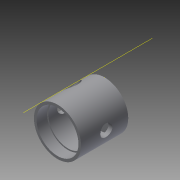
# Autodesk Inventor part: Piston
Saved by Autodesk Inventor 2015 (Build 190159000, 159)
## iProperties
Created: 2016-02-14
Part Number: Piston
Material: Generic
Document SubType Name: Modeling
Designer: Owner
Density: 1 g/cm^3
Appearance: Default
Author: Owner
Autodesk Inventor part; units mm, degrees
ref_plane "YZ Plane" through (0, 0, 0) normal (1, 0, 0) x (0, 1, 0)
ref_plane "XZ Plane" through (0, 0, 0) normal (0, 1, 0) x (-1, 0, 0)
ref_plane "XY Plane" through (0, 0, 0) normal (0, 0, 1) x (1, 0, 0)
sketch "Sketch1" plane through (0, 0, 0) normal (0, 0, 1) x (1, 0, 0)
  circle A0 centre (0, 0) radius 6.858
  dimension "d0" = 13.716
  constraints: 1 centre point, 1 coincident
  measures "d0" diameter of A0
extrude "Extrusion1" add sketch "Sketch1" along normal blind 13.716
hole "Hole1" at (0, 0, 13.716) direction (0, 0, -1) diameter 12.192 depth 3.048
hole "Hole2" at (0, 0, 10.668) direction (0, 0, -1) diameter 11.43 depth 9.144
sketch "Sketch2" plane through (0, 0, 0) normal (1, 0, 0) x (0, 1, 0)
  line L0 (0, 0) -> (0, 6.35)
  circle A0 centre (0, 6.35) radius 1.7399
  dimension "d21" = 6.35
  dimension "d22" = 3.4798
  constraints: 2 end point, 1 centre point, 1 coincident, 1 vertical
  measures "d21" distance of L0.start L0.end
  measures "d22" diameter of A0
extrude "Extrusion2" cut sketch "Sketch2" along normal through all both and the other way through all
sketch "Sketch3" plane through (0, 0, 0) normal (0, 0, -1) x (-1, 0, 0)
  line L0 (0, 0) -> (4.8942, 4.8942)
  line L1 (0, 0) -> (0, 6.9215) construction
  constraints: 4 end point, 1 vertical
sketch "Sketch4" plane through (0, 0, 0) normal (0, 1, 0) x (-1, 0, 0)
  point P0 (0, 0)
ref_plane "Work Plane1" through (-4.8942, 4.8942, 0) normal (-0.7071, 0.7071, 0) x (-0.7071, -0.7071, 0)
sketch "Sketch5" plane through (-4.8942, 4.8942, 0) normal (-0.7071, 0.7071, 0) x (-0.7071, -0.7071, 0)
  line L0 (0, 0) -> (0, 5.08)
  circle A0 centre (0, 5.08) radius 2.54
  dimension "d25" = 5.08
  dimension "d26" = 5.08
  constraints: 2 end point, 1 centre point, 1 coincident, 1 vertical
  measures "d25" distance of L0.start L0.end
  measures "d26" diameter of A0
extrude "Extrusion3" cut sketch "Sketch5" against normal up to next
body "Solid1"
